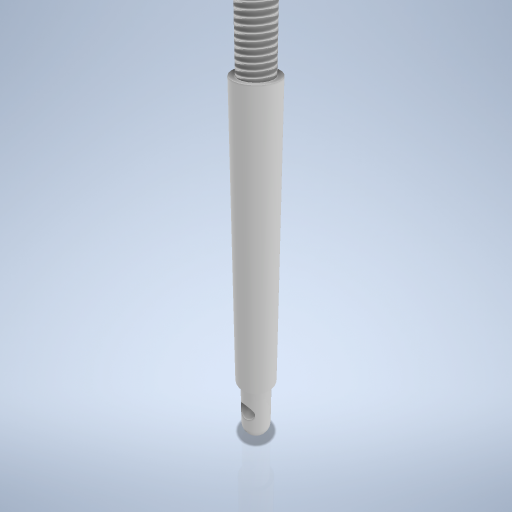
# Autodesk Inventor part: 19_2
Saved by Autodesk Inventor 2024.2 (Build 282272000, 272)
## iProperties
Created: 2024-05-15
Part Number: 19_2
Material: Generisch
Document SubType Name: Modeling
Designer: Fabri
Density: 1 g/cm^3
Appearance: Vorgabe
Author: Fabri
Autodesk Inventor part; units mm, degrees
ref_plane "YZ Plane" through (0, 0, 0) normal (1, 0, 0) x (0, 1, 0)
ref_plane "XY Plane" through (0, 0, 0) normal (0, 0, 1) x (1, 0, 0)
sketch "Skizze1" plane through (0, 0, 0) normal (0, 1, 0) x (-1, 0, 0)
  line L0 (0, 0) -> (1.5, 0)
  line L1 (1.5, 0) -> (1.5, -6.5)
  line L2 (1.5, -6.5) -> (2, -6.5)
  line L3 (2, -6.5) -> (2, -36.5)
  line L4 (0, 0) -> (0, -44)
  line L5 (2, -36.5) -> (1.5, -36.5)
  line L6 (1.5, -36.5) -> (1.5, -42.5)
  arc A0 (0, -44) -> (1.5, -42.5) centre (0, -42.5) ccw
  point P0 (0, -26.7554)
  dimension "d0" = 6.5
  dimension "d1" = 3
  dimension "d2" = 4
  dimension "d5" = 30
  dimension "d6" = 0.5
  dimension "d7" = 6
  constraints: 14 end point, 4 perpendicular, 2 horizontal, 2 point on circle, 2 vertical alignment, 1 centre point, 1 point on line, 1 tangent
  measures "d0" distance from line of L2.end L0
  measures "d1" diameter of L1 L4
  measures "d2" diameter of L3 point (0, -26.755)
  measures "d5" distance of L2.end L3.end
  measures "d6" distance of L3.end L5.end
  measures "d7" distance of L5.end L6.end
revolve "Umdrehung1" add sketch "Skizze1" angle 360 about axis through (0, 0, 0) along (0, 0, -1)
thread "Gewinde1" size "M3x0.5" class "6g" standard "ISO Metric profile" length 18
ref_plane "Arbeitsebene1" through (0, 1.75, 0) normal (0, 1, 0) x (-1, 0, 0)
sketch "Skizze2" plane through (0, 1.75, 0) normal (0, 1, 0) x (-1, 0, 0)
  line L0 (-2, -36.5) -> (2, -36.5) projected
  point P0 (0, 0)
  point P1 (0, -40)
  dimension "d13" = 3.5
  constraints: 1 vertical alignment
  measures "d13" distance from line of L0 point (0, -40)
hole "Bohrung1" at (0, 1.75, -40) direction (0, -1, 0) diameter 2 end through all
